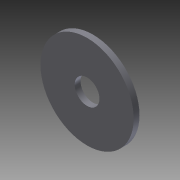
# Autodesk Inventor part: Bearing Washer
Saved by Autodesk Inventor 2014 SP1 (Build 180222100, 222)
## iProperties
Created: 2012-03-30
Part Number: Bearing Washer
Material: Steel
Document SubType Name: Modeling
Designer: Moses
Mass: 5.86773 g
Surface Area: 11.0208 cm^2
Volume: 0.747482 cm^3
Density: 7.85 g/cm^3
Appearance: Steel
Author: Moses
Autodesk Inventor part; units mm, degrees
ref_plane "YZ Plane" through (0, 0, 0) normal (1, 0, 0) x (0, 1, 0)
ref_plane "XZ Plane" through (0, 0, 0) normal (0, 1, 0) x (-1, 0, 0)
ref_plane "XY Plane" through (0, 0, 0) normal (0, 0, 1) x (1, 0, 0)
sketch "Sketch1" plane through (0, 0, 0) normal (0, 0, 1) x (1, 0, 0)
  circle A0 centre (0, 0) radius 3.3782
  circle A1 centre (0, 0) radius 12.7
  dimension "d0" = 6.7564
  dimension "d1" = 25.4
  constraints: 2 centre point, 2 coincident
  measures "d0" diameter of A0
  measures "d1" diameter of A1
extrude "Extrusion1" add sketch "Sketch1" along normal blind 1.5875
body "Solid1"
